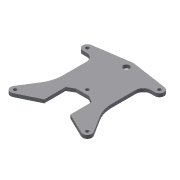
# Autodesk Inventor part: Corpo_Suporte_Cabos
Saved by Autodesk Inventor 2018 (Build 220112000, 112)
## iProperties
Created: 2021-04-27
Part Number: Corpo_Suporte_Cabos
Material: Generic
Document SubType Name: Modeling
Designer: l01767
Density: 1 g/cm^3
Appearance: Default
Author: l01767
Autodesk Inventor part; units mm, degrees
ref_plane "YZ Plane" through (0, 0, 0) normal (1, 0, 0) x (0, 1, 0)
ref_plane "XZ Plane" through (0, 0, 0) normal (0, 1, 0) x (-1, 0, 0)
ref_plane "XY Plane" through (0, 0, 0) normal (0, 0, 1) x (1, 0, 0)
sketch "Sketch1" plane through (0, 0, 0) normal (0, 0, 1) x (1, 0, 0)
  circle A0 centre (0, 0) radius 20
  circle A1 centre (-235, -20) radius 11
  line L0 (0, 0) -> (0, -376)
  line L1 (-235, -20) -> (0, -20) construction
  circle A2 centre (235, -20) radius 11
  circle A3 centre (-235, -490) radius 11
  circle A4 centre (235, -490) radius 11
  circle A5 centre (0, -255) radius 11
  arc A6 (-260.3868, -474.0154) -> (-221.9737, -517.0243) centre (-235, -490) ccw
  line L2 (-260.3868, -474.0154) -> (-191.746, -365)
  arc A7 (-239.44, 9.6696) -> (-235, -50) centre (-235, -20) ccw
  line L3 (0, -255) -> (-167.3395, -255) construction
  line L4 (235, -490) -> (-235, -490) construction
  line L5 (-221.9737, -517.0243) -> (-85, -451)
  line L6 (-85, -451) -> (-85, -311)
  line L7 (-239.44, 9.6696) -> (-6.66, 44.5044)
  arc A8 (0, 45) -> (-6.66, 44.5044) centre (0, 0) ccw
  arc A9 (-191.746, -365) -> (-160, -255) centre (-366.4481, -255) ccw
  line L8 (-235, -50) -> (-210, -50)
  line L9 (-160, -100) -> (-160, -255)
  arc A10 (-160, -100) -> (-210, -50) centre (-210, -100) ccw
  line L10 (0, 0) -> (0, 45) construction
  line L11 (235, -20) -> (0, -20) construction
  arc A11 (221.9737, -517.0243) -> (260.3868, -474.0154) centre (235, -490) ccw
  line L12 (260.3868, -474.0154) -> (191.746, -365)
  arc A12 (235, -50) -> (239.44, 9.6696) centre (235, -20) ccw
  line L13 (0, -255) -> (167.3395, -255) construction
  line L14 (-235, -490) -> (235, -490) construction
  line L15 (221.9737, -517.0243) -> (85, -451)
  line L16 (85, -451) -> (85, -311)
  line L17 (239.44, 9.6696) -> (6.66, 44.5044)
  arc A13 (160, -255) -> (191.746, -365) centre (366.4481, -255) ccw
  line L18 (235, -50) -> (210, -50)
  line L19 (160, -100) -> (160, -255)
  arc A14 (210, -50) -> (160, -100) centre (210, -100) ccw
  arc A15 (6.66, 44.5044) -> (0, 45) centre (0, 0) ccw
  line L20 (85, -311) -> (41.6987, -286)
  line L21 (41.6987, -286) -> (0, -286)
  line L22 (-85, -311) -> (-41.6987, -286)
  line L23 (-41.6987, -286) -> (0, -286)
  point P0 (0, -266)
  point P1 (0, 20)
  dimension "d0" = 40
  dimension "d12" = 22
  dimension "d1" = 22
  dimension "d2" = 235
  dimension "d5" = 470
  dimension "d8" = 470
  dimension "d11" = 20
  dimension "d13" = 235
  dimension "d14" = 30
  dimension "d15" = 30
  dimension "d17" = 140
  dimension "d18" = 110
  dimension "d19" = 50
  dimension "d21" = 20
  dimension "d23" = 75
  dimension "d24" = 25
  dimension "d27" = 60
  dimension "d28" = 75
  dimension "d29" = 25
  constraints: 46 end point, 20 point on circle, 19 symmetric about line, 14 centre point, 9 tangent, 7 point on line, 5 coincident, 5 horizontal, 5 vertical, 2 vertical alignment, 1 collinear, 1 perpendicular, 18 other
  measures "d1" diameter of A1
  measures "d2" horizontal distance of L0.start L1.start
  measures "d5" distance of L1.start A2.centre
  measures "d8" distance of L1.start A3.centre
  measures "d11" vertical distance of L0.start L1.start
  measures "d13" horizontal distance of A2.centre L3.start
  measures "d14" radius of A6
  measures "d15" radius of A7
  measures "d17" distance of L5.end L6.end
  measures "d18" vertical distance of L2.end L9.end
  measures "d19" radius of A10
  measures "d21" distance of L21.end point (0, -266)
  measures "d23" distance from line of L1.start L9
  measures "d24" distance of point (0, 20) L10.end
  measures "d27" angle of L6 L22
  measures "d28" distance between parallel lines of L9 L6
  measures "d29" distance from line of L21 L16.end
extrude "Extrusion1" add sketch "Sketch1" along normal mid plane 22.22
equation "\"d5\" = 2 * d2"
equation "\"d8\" = 2 * d2"
equation "\"d13\" = d2"
body "Solid1"
